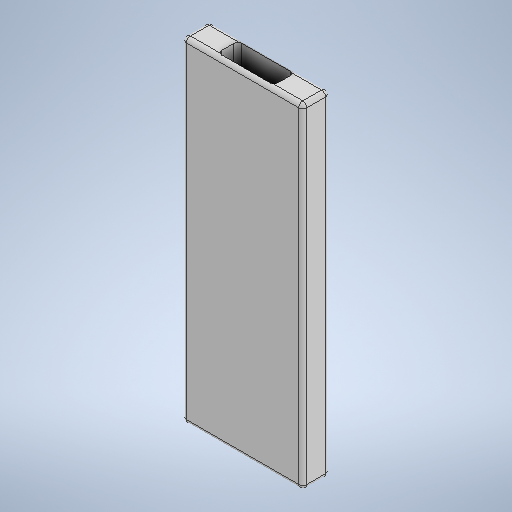
# Autodesk Inventor part: OTOSGuard
Saved by Autodesk Inventor 2025.2 (Build 292293000, 293)
## iProperties
Created: 2025-01-05
Part Number: OTOSGuard
Material: Generic
Document SubType Name: Modeling
Designer: dcfam
Density: 1 g/cm^3
Appearance: Default
Author: dcfam
Autodesk Inventor part; units mm, degrees
ref_plane "YZ Plane" through (0, 0, 0) normal (1, 0, 0) x (0, 1, 0)
ref_plane "XZ Plane" through (0, 0, 0) normal (0, 1, 0) x (-1, 0, 0)
ref_plane "XY Plane" through (0, 0, 0) normal (0, 0, 1) x (1, 0, 0)
sketch "Sketch1" plane through (0, 0, 0) normal (0, 0, 1) x (1, 0, 0)
  line L0 (-4.5, -12.5) -> (4.5, -12.5)
  line L1 (4.5, -12.5) -> (4.5, 12.5)
  line L2 (4.5, 12.5) -> (-4.5, 12.5)
  line L3 (-4.5, 12.5) -> (-4.5, -12.5)
  line L4 (-4.5, -12.5) -> (4.5, 12.5) construction
  line L5 (4.5, -12.5) -> (-4.5, 12.5) construction
  point P0 (0, 0)
  dimension "d0" = 9
  dimension "d1" = 25
  constraints: 12 end point, 2 midpoint, 2 parallel, 1 horizontal, 1 perpendicular
  measures "d0" distance of L2.end L1.end
  measures "d1" distance of L1.end L0.end
extrude "Extrusion1" add sketch "Sketch1" along normal blind 2
sketch "Sketch2" plane through (-4.5, -12.5, 0) normal (0, -1, 0) x (1, 0, 0)
  line L0 (4.5, 0) -> (4.5, 2) construction
  line L1 (9, 2) -> (0, 2) construction
  line L2 (0, 0) -> (0, 2) construction
  line L3 (0, 1) -> (9, 1) construction
  line L4 (2.4, 0.25) -> (6.6, 0.25)
  line L5 (6.6, 0.25) -> (6.6, 1.75)
  line L6 (6.6, 1.75) -> (2.4, 1.75)
  line L7 (2.4, 1.75) -> (2.4, 0.25)
  line L8 (2.4, 0.25) -> (6.6, 1.75) construction
  line L9 (6.6, 0.25) -> (2.4, 1.75) construction
  point P0 (4.5, 1)
  dimension "d4" = 4.2
  dimension "d5" = 1.5
  constraints: 16 end point, 5 midpoint, 2 horizontal, 2 parallel, 1 perpendicular
  measures "d4" distance of L6.end L5.end
  measures "d5" distance of L5.end L4.end
extrude "Extrusion2" cut sketch "Sketch2" against normal blind 254
fillet "Fillet1" radius 0.3 4 edges at (-2.1, 0, 0.25) (2.1, 0, 0.25) (-2.1, 0, 1.75) (2.1, 0, 1.75)
fillet "Fillet2" radius 0.3 12 edges at (4.5, 0, 0) (4.5, -12.5, 1) (4.5, 0, 2) (0, -12.5, 0) (0, -12.5, 2) (4.5, 12.5, 1) (0, 12.5, 0) (0, 12.5, 2) (-4.5, 12.5, 1) (-4.5, 0, 0) (-4.5, 0, 2) (-4.5, -12.5, 1)
body "Solid1"
